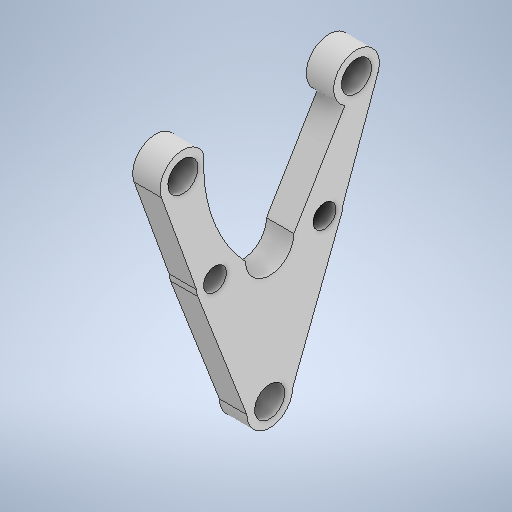
# Autodesk Inventor part: ikafly2b
Saved by Autodesk Inventor 2025 (Build 290162000, 162)
## iProperties
Created: 2024-06-13
Part Number: ikafly2b
Material: 一般
Document SubType Name: Modeling
Designer: Saigusa
Density: 1 g/cm^3
Appearance: 既定
Author: Saigusa
Autodesk Inventor part; units mm, degrees
ref_plane "YZ Plane" through (0, 0, 0) normal (1, 0, 0) x (0, 1, 0)
ref_plane "XZ Plane" through (0, 0, 0) normal (0, 1, 0) x (-1, 0, 0)
ref_plane "XY Plane" through (0, 0, 0) normal (0, 0, 1) x (1, 0, 0)
sketch "スケッチ1" plane through (0, 0, 0) normal (1, 0, 0) x (0, 1, 0)
  line L0 (0, 0) -> (0, 6)
  line L1 (0, 6) -> (0, -6)
  line L2 (0, 0) -> (11.5, 0)
  line L3 (11.5, 0) -> (11.5, 9.5)
  line L4 (11.5, 9.5) -> (11.5, -9.5)
  circle A0 centre (0, 6) radius 1.25
  circle A1 centre (0, -6) radius 1.25
  circle A2 centre (11.5, 9.5) radius 1.65
  circle A3 centre (11.5, -9.5) radius 1.65
  circle A4 centre (11.5, 9.5) radius 2.5
  circle A5 centre (11.5, -9.5) radius 2.5
  circle A6 centre (0, 0) radius 2.65
  line L5 (0, 0) -> (-14.6, 0)
  circle A7 centre (-14.6, 0) radius 1.65
  circle A8 centre (-14.6, 0) radius 2.5
  circle A9 centre (0, 6) radius 2
  circle A10 centre (0, -6) radius 2
  line L6 (0, 8) -> (10.6499, 11.851)
  line L7 (0, -8) -> (10.6499, -11.851)
  line L8 (-14.6, 0) -> (-14.6, -2.5)
  line L9 (-14.6, 0) -> (-12.1, 0) construction
  line L10 (-14.6, -2.5) -> (-14.6, 2.5)
  line L11 (-14.6, -2.5) -> (-0.7212, -7.8655)
  line L12 (-14.6, 2.5) -> (-0.7212, 7.8655)
  circle A11 centre (11.5, -9.5) radius 14.9164
  line L13 (11.5, -9.5) -> (0, 0)
  line L14 (11.5, -9.5) -> (0, -2.65)
  line L15 (14, 9.5) -> (14, 6.6979)
  circle A12 centre (11.5, -9.5) radius 16.7294
  point P0 (9.3522, -8.2206)
  point P1 (0, 2.65)
  point P2 (12.4812, 7.2006)
  dimension "d9" = 5
  dimension "d10" = 5.3
  dimension "d0" = 6
  dimension "d1" = 12
  dimension "d2" = 11.5
  dimension "d3" = 9.5
  dimension "d4" = 19
  dimension "d5" = 2.5
  dimension "d6" = 3.3
  dimension "d7" = 3.3
  dimension "d8" = 5
  dimension "d11" = 14.6
  dimension "d12" = 3.3
  dimension "d13" = 5
  dimension "d14" = 4
  dimension "d15" = 4
  dimension "d16" = 90
  constraints: 32 end point, 13 coincident, 10 centre point, 8 point on circle, 7 point on line, 4 tangent, 3 perpendicular, 2 horizontal, 1 parallel, 1 vertical, 10 other
  measures "d0" distance of L0.start L0.end
  measures "d1" distance of L0.end L1.end
  measures "d2" distance of L0.start L2.end
  measures "d3" distance of L2.end L3.end
  measures "d4" distance of L3.end L4.end
  measures "d5" diameter of A0
  measures "d6" diameter of A2
  measures "d7" diameter of A3
  measures "d8" diameter of A4
  measures "d11" distance of L5.start L5.end
  measures "d12" diameter of A7
  measures "d13" diameter of A8
  measures "d14" diameter of A9
  measures "d15" diameter of A10
  measures "d16" angle of L8 L9
extrude "押し出し2" add sketch "スケッチ1" along normal blind 3 contours A6 L5 A8 L12 A9 L0 | L0 A9 L6 A4 A12 | L14 A5 L7 A10 L1 | L1 A10 L11 A11 A6 | A11 L11 A12 A6 | A9 | A6 A12 L11 A8 L5 | A4 A12 | A10 | L14 A3 L4 A5 | A5 L13 A3 L14 | A5 L4 A3 L13 | A8 L8 A7 L5 | L5 A7 L10 A8 | L10 A7 L8 A8
